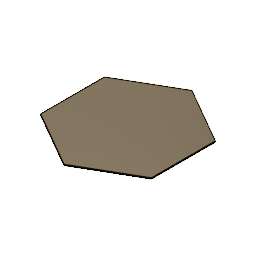
6dof v2 (Autodesk Fusion 360 design; units mm, degrees)
Autodesk Fusion 360 part; units mm, degrees
sketch "Sketch1" plane through (0, 0, 0) normal (0, 1, 0) x (1, 0, 0)
  line L0 (0, -300) -> (259.8076, -150)
  line L1 (259.8076, -150) -> (259.8076, 150)
  line L2 (259.8076, 150) -> (0, 300)
  line L3 (0, 300) -> (-259.8076, 150)
  line L4 (-259.8076, 150) -> (-259.8076, -150)
  line L5 (-259.8076, -150) -> (0, -300)
  dimension "d1" = 300
  measures "d1" distance of L0.start origin
extrude "Extrude1" add sketch "Sketch1" along normal blind 5
sketch "Sketch2" plane through (0, 5, 0) normal (0, 1, 0) x (-1, 0, 0)
  line L0 (259.8076, 150) -> (0, 300)
  line L1 (0, 300) -> (-259.8076, 150)
  line L2 (-259.8076, 150) -> (-259.8076, -150)
  line L3 (-259.8076, -150) -> (0, -300)
  line L4 (0, -300) -> (259.8076, -150)
  line L5 (259.8076, -150) -> (259.8076, 150)
